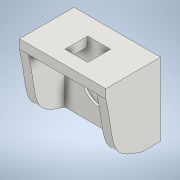
# Autodesk Inventor part: mocowanie lozyska 10-1
Saved by Autodesk Inventor 2021 (Build 250183000, 183)
## iProperties
Created: 2021-11-03
Part Number: mocowanie lozyska 10-1
Material: Generic
Document SubType Name: Modeling
Designer: Łukasz
Density: 1 g/cm^3
Appearance: Steel
Author: Łukasz
Autodesk Inventor part; units mm, degrees
ref_plane "YZ Plane" through (0, 0, 0) normal (1, 0, 0) x (0, 1, 0)
ref_plane "XZ Plane" through (0, 0, 0) normal (0, 1, 0) x (-1, 0, 0)
ref_plane "XY Plane" through (0, 0, 0) normal (0, 0, 1) x (1, 0, 0)
sketch "Sketch1" plane through (0, 0, 0) normal (0, 0, 1) x (1, 0, 0)
  circle A0 centre (0, 0) radius 11.1
  circle A1 centre (0, 0) radius 15
  line L0 (-15, 15) -> (15, 15)
  line L1 (15, 15) -> (15, -15)
  line L2 (15, -15) -> (-15, -15)
  line L3 (-15, -15) -> (-15, 15)
  dimension "d0" = 22.2
  dimension "d1" = 30
  constraints: 8 end point, 2 centre point, 2 coincident, 2 parallel, 1 horizontal, 1 perpendicular
  measures "d0" diameter of A0
  measures "d1" diameter of A1
extrude "Extrusion1" add sketch "Sketch1" along normal blind 7
sketch "Sketch2" plane through (0, 0, 7) normal (0, 0, 1) x (1, 0, 0)
  circle A0 centre (0, 0) radius 7.5
  line L0 (-15, -15) -> (15, -15) projected
  line L1 (15, -15) -> (15, 15) projected
  line L2 (15, 15) -> (-15, 15) projected
  line L3 (-15, 15) -> (-15, -15) projected
  circle A1 centre (0, 0) radius 11.1 projected
  dimension "d4" = 15
  constraints: 1 centre point, 1 coincident
  measures "d4" diameter of A0
extrude "Extrusion2" add sketch "Sketch2" along normal blind 1 contours L3 L2 L1 L0 | A1
sketch "Sketch3" plane through (0, 0, 8) normal (0, 0, 1) x (1, 0, 0)
  line L0 (15, 15) -> (-15, 15) projected
  line L1 (15, -15) -> (15, 15) projected
  line L2 (-15, 15) -> (15, 15)
  line L3 (15, 15) -> (15, 13)
  line L4 (15, 13) -> (-15, 13)
  line L5 (-15, 13) -> (-15, 15)
  point P0 (0, 0)
  dimension "d7" = 2
  constraints: 8 end point, 2 parallel, 1 horizontal, 1 perpendicular, 1 point on line
  measures "d7" distance of L2.end L3.end
extrude "Extrusion3" add sketch "Sketch3" along normal blind 10
sketch "Sketch4" plane through (-15, 15, 0) normal (0, 1, 0) x (1, 0, 0)
  line L0 (0, -18) -> (30, -18) projected
  line L1 (10, -18) -> (20, -18)
  line L2 (20, -18) -> (20, -8)
  line L3 (20, -8) -> (10, -8)
  line L4 (10, -8) -> (10, -18)
  line L5 (0, 0) -> (0, -18) projected
  point P0 (15, 0)
  dimension "d10" = 10
  dimension "d11" = 10
  dimension "d12" = 10
  constraints: 8 end point, 2 parallel, 1 horizontal, 1 perpendicular, 1 point on line
  measures "d10" distance of L3.end L2.end
  measures "d11" distance of L2.end L1.end
  measures "d12" distance between parallel lines of L5 L4
extrude "Extrusion4" cut sketch "Sketch4" against normal blind 10
sketch "Sketch5" plane through (-15, 15, 0) normal (0, 1, 0) x (1, 0, 0)
  line L0 (10, -18) -> (10, -8) projected
  line L1 (10, -8) -> (20, -8) projected
  line L2 (20, -8) -> (20, -18) projected
  line L3 (30, -18) -> (20, -18) projected
  line L4 (30, 0) -> (30, -18) projected
  line L5 (30, 0) -> (0, 0) projected
  line L6 (0, 0) -> (0, -18) projected
  line L7 (10, -18) -> (0, -18) projected
  point P0 (15, 0)
extrude "Extrusion5" add sketch "Sketch5" along normal blind 2
sketch "Sketch6" plane through (0, 0, 18) normal (0, 0, 1) x (1, 0, 0)
  line L0 (-15, 17) -> (-5, 17) projected
  line L1 (5, 13) -> (15, 13) projected
  line L2 (-15, 17) -> (15, 17)
  line L3 (15, 17) -> (15, 13)
  line L4 (15, 13) -> (-15, 13)
  line L5 (-15, 13) -> (-15, 17)
  point P0 (0, 0)
  constraints: 8 end point, 2 parallel, 1 horizontal, 1 perpendicular
extrude "Extrusion6" add sketch "Sketch6" along normal blind 6
sketch "Sketch7" plane through (15, -15, 8) normal (1, 0, 0) x (0, 0, -1)
  line L0 (0, 28) -> (-16, 28) projected
  spline S0 degree 4 poles (0, 0) (-5.902, 2.124) (-15.1303, 3.8148) (-11.9672, 10.0618) (-16, 28) knots 0 0 0 0 0 1 1 1 1 1
  line L1 (8, 0) -> (8, 32) projected
  line L2 (8, 32) -> (-16, 32) projected
  line L3 (-16, 28) -> (-16, 32) projected
  line L4 (0, 28) -> (-16, 28) projected
  line L5 (0, 0) -> (0, 28) projected
  line L6 (8, 0) -> (0, 0) projected
  point P0 (8, 15)
  point P1 (-5.2907, 1.8449)
  point P2 (-9.6455, 4.4326)
  point P3 (-12.4856, 9.1661)
  point P4 (0, 0)
  constraints: 5 other
extrude "Extrusion7" add sketch "Sketch7" along normal blind 4
sketch "Sketch8" plane through (-15, -15, 0) normal (-1, 0, 0) x (0, 0, 1)
  line L0 (8, 0) -> (0, 0) projected
  line L1 (0, 0) -> (0, 32) projected
  line L2 (0, 32) -> (24, 32) projected
  line L3 (24, 32) -> (24, 28) projected
  spline S0 degree 4 poles (24, 28) (19.9672, 10.0618) (23.1303, 3.8148) (13.902, 2.124) (8, 0) knots 0 0 0 0 0 1 1 1 1 1 projected
  point P0 (0, 15)
  constraints: 1 other
extrude "Extrusion8" add sketch "Sketch8" along normal blind 4
body "Solid1"
